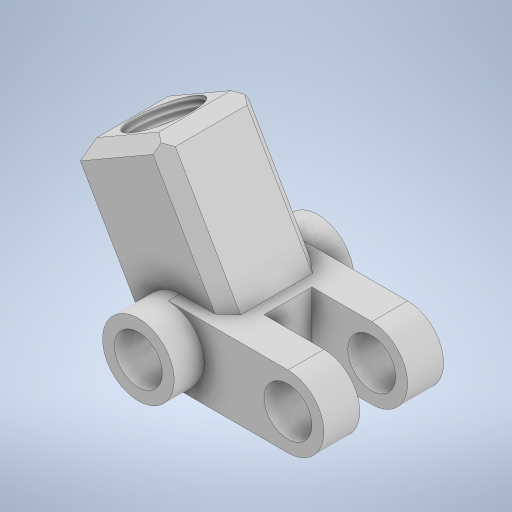
# Autodesk Inventor part: Kniehebel
Saved by Autodesk Inventor 2024 (Build 280153000, 153)
## iProperties
Created: 2023-05-12
Part Number: Kniehebel
Material: Generic
Document SubType Name: Modeling
Designer: Raj
Density: 1 g/cm^3
Appearance: Default
Author: Raj
Autodesk Inventor part; units mm, degrees
ref_plane "YZ Plane" through (0, 0, 0) normal (1, 0, 0) x (0, 1, 0)
ref_plane "XZ Plane" through (0, 0, 0) normal (0, 1, 0) x (-1, 0, 0)
sketch "Sketch1" plane through (0, 0, 0) normal (0, 1, 0) x (-1, 0, 0)
  line L0 (0, 0) -> (-20, 0) construction
  line L1 (0, 6) -> (-20, 6)
  line L2 (-20, -6) -> (0, -6)
  arc A0 (0, -6) -> (0, 6) centre (0, 0) ccw
  arc A1 (-20, 6) -> (-20, -6) centre (-20, 0) ccw
  circle A2 centre (0, 0) radius 4
  circle A3 centre (-20, 0) radius 4
  point P0 (-10, 0)
  dimension "d0" = 20
  dimension "d1" = 12
  dimension "d4" = 8
  dimension "d5" = 8
  constraints: 8 end point, 4 centre point, 4 point on circle, 4 tangent, 2 coincident, 1 horizontal, 1 midpoint, 1 parallel
  measures "d0" distance of L0.start L0.end
  measures "d1" diameter of A1
  measures "d4" diameter of A2
  measures "d5" diameter of A3
extrude "Extrusion1" add sketch "Sketch1" along normal blind 20
sketch "Sketch2" plane through (0, 0, 6) normal (0, 0, 1) x (1, 0, 0)
  line L0 (26, 0) -> (26, 20) projected
  line L1 (10, 14) -> (26, 14)
  line L2 (26, 14) -> (26, 6)
  line L3 (26, 6) -> (10, 6)
  line L4 (10, 6) -> (10, 14)
  line L5 (0, 20) -> (20, 20) projected
  point P0 (0, 0)
  dimension "d6" = 16
  dimension "d7" = 8
  dimension "d8" = 6
  constraints: 8 end point, 2 parallel, 1 horizontal, 1 perpendicular, 1 point on line
  measures "d6" distance of L1.start L1.end
  measures "d7" distance between parallel lines of L3 L1
  measures "d8" distance between parallel lines of L1 L5
extrude "Extrusion2" cut sketch "Sketch2" against normal through all
ref_plane "Work Plane1" through (0, 10, 0) normal (0, 1, 0) x (1, 0, 0)
sketch "Sketch4" plane through (0, 10, 0) normal (0, 1, 0) x (1, 0, 0)
  circle A0 centre (0, 0) radius 6
  line L0 (20, 6) -> (0, 6) projected
  circle A1 centre (0, 0) radius 4
  dimension "d12" = 8
  constraints: 2 coincident, 1 centre point, 1 horizontal, 1 vertical alignment, 1 other
  measures "d12" diameter of A1
extrude "Extrusion3" add sketch "Sketch4" along normal mid plane 30
sketch "Sketch5" plane through (0, 10, 0) normal (0, 1, 0) x (1, 0, 0)
  line L0 (-5.1962, 3) -> (-17.6962, -18.6506)
  line L1 (-3.8397, -26.6506) -> (8.6603, -5)
  line L2 (-3.8397, -26.6506) -> (-17.6962, -18.6506)
  circle A0 centre (0, 0) radius 6 projected
  line L3 (20, 6) -> (0, 6) projected
  line L4 (0, -6) -> (20, -6) projected
  point P0 (8.0829, -6)
  dimension "d17" = 120
  dimension "d18" = 25
  dimension "d20" = 120
  dimension "d22" = 25
  dimension "d24" = 13.8564
  constraints: 6 end point, 1 perpendicular, 1 point on circle, 1 tangent
  measures "d17" angle of L3 L0
  measures "d18" distance from line of point (0, 0) L2
  measures "d20" angle of L4 L1
  measures "d22" distance of L1.start L1.end
  measures "d24" horizontal distance of L1.end L0.start
extrude "Extrusion4" add sketch "Sketch5" along normal mid plane 16 contours A0 L4 L1 L2 L0
sketch "Sketch6" plane through (-3.8397, 2, 26.6506) normal (-0.5, 0, 0.8660254) x (0.8660254, 0, 0.5)
  line L0 (-16, 0) -> (-16, 16) projected
  line L1 (-16, 16) -> (0, 16) projected
  point P0 (-10, -2)
  point P1 (-8, 8)
  dimension "d27" = 8
  dimension "d28" = 8
  measures "d27" distance from line of L0 point (-8, 8)
  measures "d28" distance from line of point (-8, 8) L1
hole "Hole1" at (-10.7679, 10, 22.6506) direction (0.5, 0, -0.8660254) diameter 10.917 depth 16 tip angle 118 thread size "M12x1" class "6H" standard "ISO Metric profile"
chamfer "Chamfer1" distance 2 angle 45 6 edges at (2.1216, 2, 16.3253) (2.1216, 18, 16.3253) (-3.8397, 10, 26.6506) (-10.7679, 2, 22.6506) (-17.6962, 10, 18.6506) (-10.7679, 18, 22.6506)
body "Solid1"
